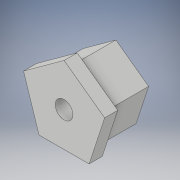
# Autodesk Inventor part: gearNotch
Saved by Autodesk Inventor 2019.1 (Build 231200000, 200)
## iProperties
Created: 2018-12-01
Part Number: gearNotch
Material: Generisch
Document SubType Name: Modeling
Designer: JochenAlt
Density: 1 g/cm^3
Appearance: Vorgabe
Author: JochenAlt
Autodesk Inventor part; units mm, degrees
ref_plane "YZ Plane" through (0, 0, 0) normal (1, 0, 0) x (0, 1, 0)
ref_plane "XZ Plane" through (0, 0, 0) normal (0, 1, 0) x (-1, 0, 0)
ref_plane "XY Plane" through (0, 0, 0) normal (0, 0, 1) x (1, 0, 0)
sketch "Skizze1" plane through (0, 0, 0) normal (0, 0, 1) x (1, 0, 0)
  circle A0 centre (0, 0) radius 3.75 construction
  line L0 (0, 3.75) -> (3.5665, 1.1588)
  line L1 (3.5665, 1.1588) -> (2.2042, -3.0338)
  line L2 (2.2042, -3.0338) -> (-2.2042, -3.0338)
  line L3 (-2.2042, -3.0338) -> (-3.5665, 1.1588)
  line L4 (-3.5665, 1.1588) -> (0, 3.75)
  circle A1 centre (0, 0) radius 5.25 construction
  line L5 (0, 5.25) -> (4.993, 1.6223)
  line L6 (4.993, 1.6223) -> (3.0859, -4.2473)
  line L7 (3.0859, -4.2473) -> (-3.0859, -4.2473)
  line L8 (-3.0859, -4.2473) -> (-4.993, 1.6223)
  line L9 (-4.993, 1.6223) -> (0, 5.25)
  circle A2 centre (0, 0) radius 1.3462
  circle A3 centre (0, 0) radius 6.5 construction
  line L10 (-6.1819, 2.0086) -> (0, 6.5)
  line L11 (0, 6.5) -> (6.1819, 2.0086)
  line L12 (6.1819, 2.0086) -> (3.8206, -5.2586)
  line L13 (3.8206, -5.2586) -> (-3.8206, -5.2586)
  line L14 (-3.8206, -5.2586) -> (-6.1819, 2.0086)
  line L15 (0, 9.1) -> (0, -9.1) construction
  circle A4 centre (0, 0) radius 4.3846 construction
  dimension "d19" = 10.5
  dimension "d20" = 13
  dimension "d21" = 7.5
  constraints: 30 end point, 7 coincident, 2 centre point, 2 parallel, 2 vertical alignment, 1 point on line, 40 other
extrude "Extrusion1" add sketch "Skizze1" along normal blind 4.4 contours L5 L6 L7 L8 L9
extrude "Extrusion2" add sketch "Skizze1" along normal blind 1.5 from surface at 4.4 contours L0 L1 L2 L3 L4 | L5 L6 L7 L8 L9
extrude "Extrusion3" add sketch "Skizze1" along normal blind 2 from surface at 5.9 contours L0 L1 L2 L3 L4 | L5 L6 L7 L8 L9 | L10 L11 L12 L13 L14
